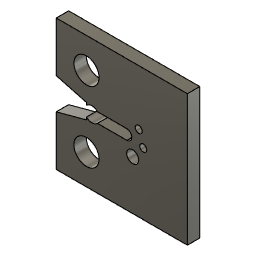
Sandia_1st_Fracture_Challenge (Autodesk Fusion 360 design; units mm, degrees)
Autodesk Fusion 360 part; units mm, degrees
sketch "Sketch1" plane through (0, 0, 0) normal (0, 0, 1) x (1, 0, 0)
  line L0 (-7.62, 16.51) -> (25.4, 16.51)
  line L1 (25.4, 16.51) -> (25.4, -16.51)
  line L2 (25.4, -16.51) -> (-7.62, -16.51)
  circle A0 centre (0, 8.89) radius 3.175
  circle A1 centre (0, -8.89) radius 3.175
  circle A2 centre (13.15, 2.61) radius 0.89
  circle A3 centre (14.29, -0.89) radius 0.89
  circle A4 centre (11.63, -4.12) radius 1.525
  line L3 (-7.62, 3.9468) -> (0, 1.905)
  line L4 (2.7588, 1.27) -> (10.16, 1.27)
  arc A5 (10.16, -1.27) -> (10.16, 1.27) centre (10.16, 0) ccw
  line L5 (10.16, -1.27) -> (2.7588, -1.27)
  arc A6 (0, -1.27) -> (2.7588, -1.27) centre (1.3794, 0) ccw
  line L6 (0, -1.27) -> (0, -1.905)
  line L7 (0, -1.905) -> (-7.62, -3.9468)
  line L8 (-7.62, -16.51) -> (-7.62, -3.9468)
  line L9 (-7.62, 3.9468) -> (-7.62, 16.51)
  line L10 (0, 110) -> (0, -80) construction
  line L11 (11.43, -80) -> (11.43, 100) construction
  line L12 (-90, 0) -> (-86.3571, 0) construction
  line L13 (-86.3571, 0) -> (70, 0) construction
  line L14 (0, 1.905) -> (0, 1.27)
  arc A7 (2.7588, 1.27) -> (0, 1.27) centre (1.3794, 0) ccw
  dimension "d1" = 6.35
  dimension "d2" = 7.62
  dimension "d3" = 7.62
  dimension "d4" = 33.02
  dimension "d5" = 1.27
  dimension "d6" = 19.05
  dimension "d10" = 15
  dimension "d11" = 1.905
  dimension "d12" = 1.905
  dimension "d14" = 7.62
  dimension "d15" = 1.78
  dimension "d16" = 1.78
  dimension "d17" = 3.05
  dimension "d18" = 12.39
  dimension "d19" = 13.77
  dimension "d20" = 11.11
  dimension "d21" = 15.62
  dimension "d22" = 12.25
  dimension "d23" = 13.9
  dimension "d24" = 33.02
  dimension "d26" = 1.875
  dimension "d27" = 15
  dimension "d28" = 2.54
  constraint horizontal L0
  constraint vertical L1
  constraint horizontal L2
  constraint vertical L8
  constraint coincident L3.start L8
  constraint horizontal L4
  constraint tangent L4 A5
  constraint parallel L4 L5
  constraint collinear L8 L9
  constraint perpendicular L2 L10
  constraint coincident origin L10
  constraint coincident A0.centre L10
  constraint coincident A1.centre L10
  constraint equal A0 A1
  constraint tangent A5 L5
  constraint perpendicular L4 L11
  constraint tangent A5 L11
  constraint horizontal L12
  constraint parallel L12 L13
  constraint coincident origin L13
  constraint coincident A5.centre L13
  constraint vertical L6
  constraint equal L4 L5
  constraint equal L3 L7
  constraint coincident A6.centre L13
  constraint equal L8 L9
  constraint coincident L10 L14.end
  constraint vertical L14
  constraint equal A6 A7
  constraint equal L6 L14
  measures "d1" diameter of A1
  measures "d2" distance of L2 A1.centre
  measures "d3" distance of L0 A0.centre
  measures "d4" distance of L0.start L0.end
  measures "d5" radius of A5
  measures "d6" distance of L9 L11
  measures "d10" angle of L7 L13
  measures "d11" distance of L3.end L13
  measures "d12" distance of L6.end L13
  measures "d14" distance of A0.centre L9
  measures "d15" diameter of A2
  measures "d16" diameter of A3
  measures "d17" diameter of A4
  measures "d18" distance of L2 A4.centre
  measures "d19" distance of L1 A4.centre
  measures "d20" distance of L1 A3.centre
  measures "d21" distance of L2 A3.centre
  measures "d22" distance of L1 A2.centre
  measures "d23" distance of L0 A2.centre
  measures "d24" distance of L0.end L1.end
  measures "d26" radius of A7
  measures "d27" angle of L3 L13
  measures "d28" distance of A6.start L14.end
extrude "Extrude1" add sketch "Sketch1" along normal mid plane 3.124
